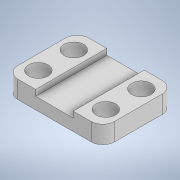
# Autodesk Inventor part: lockbelt
Saved by Autodesk Inventor 2022 (Build 260153000, 153)
## iProperties
Created: 2022-02-28
Part Number: lockbelt
Material: Genérico
Document SubType Name: Modeling
Designer: JK
Density: 1 g/cm^3
Appearance: Valor por defecto
Author: JK
Autodesk Inventor part; units mm, degrees
ref_plane "YZ Plane" through (0, 0, 0) normal (1, 0, 0) x (0, 1, 0)
ref_plane "XZ Plane" through (0, 0, 0) normal (0, 1, 0) x (-1, 0, 0)
ref_plane "XY Plane" through (0, 0, 0) normal (0, 0, 1) x (1, 0, 0)
sketch "Boceto1" plane through (0, 0, 0) normal (0, 1, 0) x (-1, 0, 0)
  line L0 (-3.175, 6) -> (3.175, 6)
  line L1 (3.175, 6) -> (3.175, -6)
  line L2 (3.175, -6) -> (-3.175, -6)
  line L3 (-3.175, -6) -> (-3.175, 6)
  line L4 (-3.175, 6) -> (3.175, -6) construction
  line L5 (3.175, 6) -> (-3.175, -6) construction
  line L6 (8.175, 6) -> (-8.175, 6)
  line L7 (-8.175, 6) -> (-8.175, -6)
  line L8 (-8.175, -6) -> (8.175, -6)
  line L9 (8.175, -6) -> (8.175, 6)
  circle A0 centre (5.7194, 3) radius 1.65
  circle A1 centre (5.7194, -3) radius 1.65
  circle A2 centre (-5.6782, 3) radius 1.65
  circle A3 centre (-5.6782, -3) radius 1.65
  point P0 (0, 0)
  dimension "d0" = 6.35
  dimension "d1" = 12
  dimension "d2" = 5
  dimension "d3" = 5
  dimension "d4" = 3.3
  dimension "d5" = 3
  dimension "d6" = 3
  constraints: 20 end point, 4 centre point, 4 parallel, 3 equal radius, 2 horizontal, 2 horizontal alignment, 2 midpoint, 2 perpendicular, 2 vertical alignment, 1 collinear
  measures "d0" distance of L0.start L0.end
  measures "d1" distance of L0.end L1.end
  measures "d2" distance between parallel lines of L9 L1
  measures "d3" distance between parallel lines of L3 L7
  measures "d4" diameter of A0
  measures "d5" distance from line of L6 A0.centre
  measures "d6" distance from line of L8 A1.centre
extrude "Extrusión1" add sketch "Boceto1" along normal blind 3
sketch "Boceto2" plane through (0, 3, 0) normal (0, 1, 0) x (1, 0, 0)
  line L0 (8.175, 6) -> (-8.175, 6) projected
  line L1 (3.175, -6) -> (-3.175, -6)
  line L2 (-3.175, -6) -> (-3.175, 6)
  line L3 (-3.175, 6) -> (3.175, 6)
  line L4 (3.175, 6) -> (3.175, -6)
  line L5 (3.175, -6) -> (-3.175, 6) construction
  line L6 (-3.175, -6) -> (3.175, 6) construction
  point P0 (0, 0)
  dimension "d9" = 6.35
  constraints: 12 end point, 2 midpoint, 2 parallel, 1 horizontal, 1 perpendicular, 1 point on line
  measures "d9" distance between parallel lines of L2 L4
extrude "Extrusión2" cut sketch "Boceto2" against normal blind 1
fillet "Empalme1" radius 2 4 edges at (-8.175, 1.5, 6) (8.175, 1.5, 6) (8.175, 1.5, -6) (-8.175, 1.5, -6)
